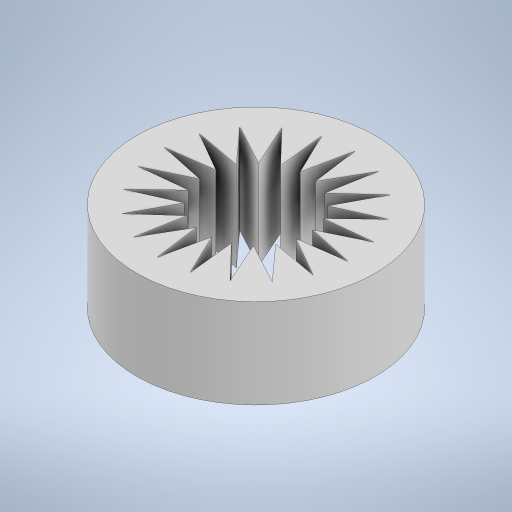
# Autodesk Inventor part: flipper_robot_v2_servo_top_adapter
Saved by Autodesk Inventor 2023.1 (Build 271208000, 208)
## iProperties
Created: 2025-10-21
Part Number: flipper_robot_v2_servo_top_adapter
Material: Generic
Document SubType Name: Modeling
Designer: Lars
Density: 1 g/cm^3
Appearance: Default
Author: Lars
Autodesk Inventor part; units mm, degrees
ref_plane "YZ Plane" through (0, 0, 0) normal (1, 0, 0) x (0, 1, 0)
ref_plane "XZ Plane" through (0, 0, 0) normal (0, 1, 0) x (-1, 0, 0)
ref_plane "XY Plane" through (0, 0, 0) normal (0, 0, 1) x (1, 0, 0)
sketch "Sketch1" plane through (0, 0, 0) normal (0, 1, 0) x (-1, 0, 0)
  circle A0 centre (0, 0) radius 3.2 construction
  circle A1 centre (0, 0) radius 1.7 construction
  line L0 (0, 0) -> (1.4858, -0.8261) construction
  line L1 (0, 0) -> (1.1578, -1.2448) construction
  line L2 (1.4858, -0.8261) -> (1.1578, -1.2448) construction
  line L3 (1.4858, -0.8261) -> (2.5191, -1.9733)
  line L4 (1.1578, -1.2448) -> (2.5191, -1.9733)
  line L5 (1.6683, -0.3265) -> (3.0056, -1.0983)
  line L6 (1.4858, -0.8261) -> (3.0056, -1.0983)
  line L7 (1.6876, 0.205) -> (3.1979, -0.1158)
  line L8 (1.6683, -0.3265) -> (3.1979, -0.1158)
  line L9 (1.5416, 0.7165) -> (3.0772, 0.8781)
  line L10 (1.6876, 0.205) -> (3.0772, 0.8781)
  line L11 (1.2448, 1.1578) -> (2.6552, 1.786)
  line L12 (1.5416, 0.7165) -> (2.6552, 1.786)
  line L13 (0.8261, 1.4858) -> (1.9733, 2.5191)
  line L14 (1.2448, 1.1578) -> (1.9733, 2.5191)
  line L15 (0.3265, 1.6683) -> (1.0983, 3.0056)
  line L16 (0.8261, 1.4858) -> (1.0983, 3.0056)
  line L17 (-0.205, 1.6876) -> (0.1158, 3.1979)
  line L18 (0.3265, 1.6683) -> (0.1158, 3.1979)
  line L19 (-0.7165, 1.5416) -> (-0.8781, 3.0772)
  line L20 (-0.205, 1.6876) -> (-0.8781, 3.0772)
  line L21 (-1.1578, 1.2448) -> (-1.786, 2.6552)
  line L22 (-0.7165, 1.5416) -> (-1.786, 2.6552)
  line L23 (-1.4858, 0.8261) -> (-2.5191, 1.9733)
  line L24 (-1.1578, 1.2448) -> (-2.5191, 1.9733)
  line L25 (-1.6683, 0.3265) -> (-3.0056, 1.0983)
  line L26 (-1.4858, 0.8261) -> (-3.0056, 1.0983)
  line L27 (-1.6876, -0.205) -> (-3.1979, 0.1158)
  line L28 (-1.6683, 0.3265) -> (-3.1979, 0.1158)
  line L29 (-1.5416, -0.7165) -> (-3.0772, -0.8781)
  line L30 (-1.6876, -0.205) -> (-3.0772, -0.8781)
  line L31 (-1.2448, -1.1578) -> (-2.6552, -1.786)
  line L32 (-1.5416, -0.7165) -> (-2.6552, -1.786)
  line L33 (-0.8261, -1.4858) -> (-1.9733, -2.5191)
  line L34 (-1.2448, -1.1578) -> (-1.9733, -2.5191)
  line L35 (-0.3265, -1.6683) -> (-1.0983, -3.0056)
  line L36 (-0.8261, -1.4858) -> (-1.0983, -3.0056)
  line L37 (0.205, -1.6876) -> (-0.1158, -3.1979)
  line L38 (-0.3265, -1.6683) -> (-0.1158, -3.1979)
  line L39 (0.7165, -1.5416) -> (0.8781, -3.0772)
  line L40 (0.205, -1.6876) -> (0.8781, -3.0772)
  line L41 (1.1578, -1.2448) -> (1.786, -2.6552)
  line L42 (0.7165, -1.5416) -> (1.786, -2.6552)
  circle A2 centre (0, 0) radius 4
  point P0 (1.6876, 0.205)
  point P1 (1.5416, 0.7165)
  point P2 (1.2448, 1.1578)
  point P3 (0.8261, 1.4858)
  point P4 (-0.7165, 1.5416)
  point P5 (-1.1578, 1.2448)
  point P6 (-1.4858, 0.8261)
  point P7 (-1.6683, 0.3265)
  point P8 (-1.6876, -0.205)
  point P9 (-1.5416, -0.7165)
  point P10 (-0.8261, -1.4858)
  point P11 (0.205, -1.6876)
  point P12 (0.7165, -1.5416)
  point P13 (1.1578, -1.2448)
  dimension "d1" = 1.5
  dimension "d5" = 18
  dimension "d6" = 0.4187
  dimension "d9" = 360
  dimension "d13" = 8
  dimension "d16" = 3.4
  constraints: 86 end point, 2 centre point, 2 coincident, 2 point on circle, 1 equal length, 104 other
  measures "d5" angle of L1 L0
  measures "d6" vertical distance of L0.end L1.end
  measures "d13" diameter of A2
  measures "d16" diameter of A1
extrude "Extrusion2" add sketch "Sketch1" along normal blind 3
body "Solid2"
